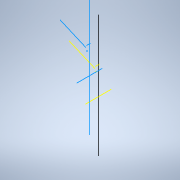
# Autodesk Inventor part: Hopper
Saved by Autodesk Inventor 2021 (Build 250183000, 183)
## iProperties
Created: 2021-03-12
Part Number: Hopper
Material: Generic
Document SubType Name: Modeling
Designer: deli
Density: 1 g/cm^3
Appearance: Default
Author: deli
Autodesk Inventor part; units mm, degrees
ref_plane "YZ Plane" through (0, 0, 0) normal (1, 0, 0) x (0, 1, 0)
ref_plane "XZ Plane" through (0, 0, 0) normal (0, 1, 0) x (-1, 0, 0)
ref_plane "XY Plane" through (0, 0, 0) normal (0, 0, 1) x (1, 0, 0)
sketch "Sketch1" plane through (0, 0, 0) normal (1, 0, 0) x (0, 1, 0)
  line L0 (19.3229, -9.5384) -> (-84.6771, -9.5384)
  line L1 (-84.6771, 38.4616) -> (-84.6771, -9.5384)
  line L2 (19.3229, -2.6574) -> (19.3229, -9.5384)
  line L3 (19.3229, -2.6574) -> (14.2746, 4.5523)
  line L4 (-84.6771, -5.5384) -> (-17.729, -5.5384)
  arc A0 (-17.729, -5.5384) -> (14.2746, 4.5523) centre (-17.729, 50.2581) ccw
  line L5 (14.2746, 4.5523) -> (151.8922, 100.9131)
  point P0 (0, 0)
  dimension "d1" = 4
  constraints: 12 end point, 2 point on circle, 2 tangent, 1 centre point, 1 horizontal, 1 point on line, 2 other
  measures "d1" distance between parallel lines of L4 L0
extrude "Extrusion1" add sketch "Sketch1" along normal blind 152.4
body "Solid1"
